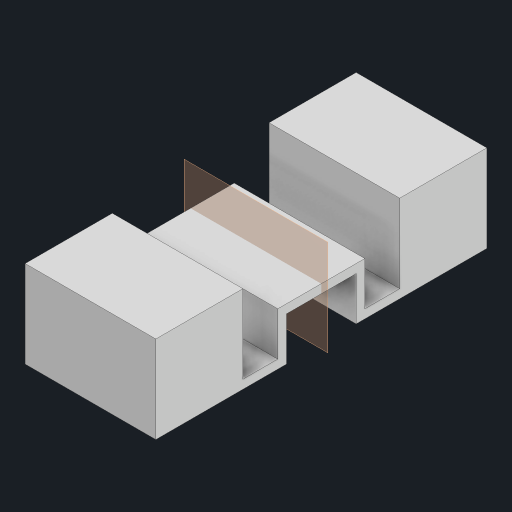
# Autodesk Inventor part: carriage_slider_top
Saved by Autodesk Inventor 2024 (Build 280153000, 153)
## iProperties
Created: 2024-06-23
Part Number: carriage_slider_top
Material: Generic
Document SubType Name: Modeling
Designer: mihir
Density: 1 g/cm^3
Appearance: Default
Author: mihir
Autodesk Inventor part; units mm, degrees
ref_plane "YZ Plane" through (0, 0, 0) normal (1, 0, 0) x (0, 1, 0)
ref_plane "XZ Plane" through (0, 0, 0) normal (0, 1, 0) x (-1, 0, 0)
ref_plane "XY Plane" through (0, 0, 0) normal (0, 0, 1) x (1, 0, 0)
sketch "Sketch1" plane through (0, 0, 0) normal (0, 1, 0) x (-1, 0, 0)
  line L0 (0, 0) -> (30, 0)
  line L1 (30, 0) -> (30, -76)
  line L2 (30, -76) -> (0, -76)
  line L3 (0, -76) -> (0, 0)
  dimension "d0" = 76
  dimension "d1" = 30
  constraints: 8 end point, 2 parallel, 1 horizontal, 1 perpendicular
  measures "d0" distance of L2.end L0.start
  measures "d1" distance of L0.start L0.end
extrude "Extrusion1" add sketch "Sketch1" along normal blind 2
sketch "Sketch2" plane through (-30, 0, 0) normal (0, 0, 1) x (1, 0, 0)
  line L0 (30, 0) -> (0, 0) projected
  line L1 (0, 0) -> (30, 0)
  line L2 (30, 0) -> (30, 20)
  line L3 (30, 20) -> (0, 20)
  line L4 (0, 20) -> (0, 0)
  line L5 (30, 0) -> (30, 2) projected
  dimension "d4" = 20
  constraints: 8 end point, 2 parallel, 1 collinear, 1 horizontal, 1 perpendicular
  measures "d4" distance of L3.end L0.end
extrude "Extrusion2" add sketch "Sketch2" against normal blind 20
sketch "Sketch3" plane through (0, 0, 0) normal (0, -1, 0) x (1, 0, 0)
  line L0 (-5, -10) -> (-25, -10)
  line L1 (-25, -10) -> (-25, -15)
  line L2 (-25, -15) -> (-5, -15)
  line L3 (-5, -15) -> (-5, -10)
  line L4 (-30, 0) -> (0, 0) projected
  line L5 (-30, -76) -> (-30, 0) projected
  dimension "d7" = 20
  dimension "d8" = 5
  dimension "d9" = 15
  dimension "d10" = 5
  constraints: 8 end point, 2 parallel, 1 horizontal, 1 perpendicular
  measures "d7" distance of L0.start L0.end
  measures "d8" distance of L2.end L0.start
  measures "d9" distance between parallel lines of L4 L2
  measures "d10" distance between parallel lines of L5 L1
revolve "Revolution1" cut sketch "Sketch3" angle 360 about axis through (-5, 0, -10) along (-1, 0, 0)
ref_plane "Work Plane1" through (-30, 0, -38) normal (0, 0, 1) x (1, 0, 0)
sketch "Sketch4" plane through (0, 0, 0) normal (0, -1, 0) x (1, 0, 0)
  line L0 (0, 0) -> (0, -76) construction
  line L1 (0, -38) -> (-30, -38) construction
  line L2 (-30, -76) -> (-30, -20) construction
  line L3 (-30, -46) -> (0, -46)
  line L4 (0, -46) -> (0, -30)
  line L5 (0, -30) -> (-30, -30)
  line L6 (-30, -30) -> (-30, -46)
  line L7 (-30, -46) -> (0, -30) construction
  line L8 (0, -46) -> (-30, -30) construction
  point P0 (-15, -38)
  dimension "d12" = 16
  constraints: 14 end point, 4 midpoint, 3 parallel, 1 collinear, 1 horizontal, 1 perpendicular, 1 point on line
  measures "d12" distance between parallel lines of L3 L5
extrude "Extrusion3" cut sketch "Sketch4" against normal up to surface (2 mm away)
sketch "Sketch5" plane through (0, 0, 0) normal (1, 0, 0) x (0, 0, -1)
  line L0 (30, 0) -> (30, 2) projected
  line L1 (30, 0) -> (28, 0)
  line L2 (28, 0) -> (28, 10)
  line L3 (28, 10) -> (30, 10)
  line L4 (30, 10) -> (30, 0)
  line L5 (28, 10) -> (38, 10)
  line L6 (38, 10) -> (38, 12)
  line L7 (38, 12) -> (28, 12)
  line L8 (28, 12) -> (28, 10)
  point P0 (0, 0)
  dimension "d15" = 2
  dimension "d16" = 10
  dimension "d17" = 2
  dimension "d18" = 10
  constraints: 16 end point, 4 parallel, 2 horizontal, 2 perpendicular
  measures "d15" distance of L2.end L3.end
  measures "d16" distance of L3.end L0.start
  measures "d17" distance of L5.end L6.end
  measures "d18" distance of L6.end L7.end
extrude "Extrusion4" add sketch "Sketch5" against normal up to surface (30 mm away)
sketch "Sketch6" plane through (0, 0, 0) normal (0, -1, 0) x (1, 0, 0)
  line L0 (-5, -15) -> (-25, -15) construction
  line L1 (-30, -30) -> (0, -30) construction
  line L2 (-5, -15) -> (-25, -15) construction
  line L3 (-25, -15) -> (-25, -30) construction
  line L4 (-25, -30) -> (-5, -30) construction
  line L5 (-5, -30) -> (-5, -15) construction
  line L6 (-25, -15) -> (-25, -5) construction
  line L7 (-5, -22.5) -> (-25, -22.5) construction
  line L8 (-20, -22.5) -> (-10, -22.5) construction
  point P0 (0, 0)
  point P1 (-15, -22.5)
  dimension "d21" = 10
  constraints: 12 end point, 4 midpoint, 2 horizontal, 2 parallel, 1 collinear, 1 perpendicular, 1 point on line
  measures "d21" distance of L8.start L8.end
hole "Hole1" at (-10, 0, -22.5) at (-20, 0, -22.5) direction (0, 1, 0) diameter 1 depth 2 tip angle 118
mirror "Mirror1" about plane through (-30, 0, -38) normal (0, 0, 1) of "Extrusion2", "Revolution1", "Extrusion4", "Hole1"
equation "\"d1\" = slider_top_width"
equation "\"d2\" = slider_top_thickness"
equation "\"d4\" = slider_top_height"
equation "\"d5\" = 2 * bearing_dist - bearing_diameter"
equation "\"d7\" = bearing_length"
equation "\"d8\" = 0.5 * bearing_diameter"
equation "\"d9\" = bearing_dist"
equation "\"d10\" = bearing_dist - bearing_diameter"
equation "\"d13\" = 2 * bearing_dist - bearing_diameter"
equation "\"d16\" = cutout_height"
equation "\"d21\" = screw_dist"
equation "\"d22\" = screw_diameter"
equation "\"slider_top_width\" = 30"
equation "\"slider_top_height\" = 20"
equation "\"slider_top_thickness\" = 2"
equation "\"bearing_length\" = 20"
equation "\"bearing_diameter\" = 10"
equation "\"bearing_dist\" = 15"
equation "\"lead_screw_outer_diameter\" = 12"
equation "\"cutout_height\" = 10"
equation "\"screw_dist\" = 10"
equation "\"screw_diameter\" = 1"
body "Solid1"
